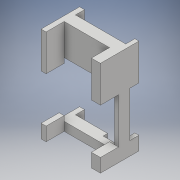
# Autodesk Inventor part: 120mmLaptopStand-Right
Saved by Autodesk Inventor 2017 (Build 210142000, 142)
## iProperties
Created: 2016-09-14
Part Number: 120mmLaptopStand-Right
Material: Generic
Document SubType Name: Modeling
Designer: Schmidty15
Density: 1 g/cm^3
Appearance: Default
Author: Schmidty15
Autodesk Inventor part; units mm, degrees
ref_plane "YZ Plane" through (0, 0, 0) normal (1, 0, 0) x (0, 1, 0)
ref_plane "XZ Plane" through (0, 0, 0) normal (0, 1, 0) x (-1, 0, 0)
ref_plane "XY Plane" through (0, 0, 0) normal (0, 0, 1) x (1, 0, 0)
sketch "Sketch1" plane through (0, 0, 0) normal (0, 1, 0) x (-1, 0, 0)
  point P0 (0, 0)
sketch "Sketch2" plane through (0, 0, 0) normal (0, 1, 0) x (-1, 0, 0)
  line L0 (0, 0) -> (-160, 0)
  line L1 (-160, 0) -> (-160, 210)
  line L2 (-160, 210) -> (0, 210)
  line L3 (0, 210) -> (0, 0)
  dimension "d0" = 160
  dimension "d1" = 210
  constraints: 8 end point, 2 parallel, 1 horizontal, 1 perpendicular
  measures "d0" distance of L1.end L2.end
  measures "d1" distance of L0.end L1.end
extrude "Extrusion1" add sketch "Sketch2" against normal blind 55
sketch "Sketch3" plane through (0, 0, 0) normal (-1, 0, 0) x (0, 0, 1)
  line L0 (0, 0) -> (0, -55) projected
  line L1 (0, 0) -> (9, 0)
  line L2 (9, 0) -> (9, -10)
  line L3 (9, -10) -> (0, -10)
  line L4 (0, -10) -> (0, 0)
  line L5 (0, 0) -> (210, 0) projected
  line L6 (9, -10) -> (131, -10)
  line L7 (131, -10) -> (131, 0)
  line L8 (131, 0) -> (9, 0)
  line L9 (9, 0) -> (9, -10)
  dimension "d4" = 9
  dimension "d5" = 10
  dimension "d6" = 122
  constraints: 16 end point, 4 parallel, 2 horizontal, 2 perpendicular, 1 point on line
  measures "d4" distance of L2.end L3.end
  measures "d5" distance of L1.end L2.end
  measures "d6" distance of L8.end L7.end
extrude "Extrusion2" cut sketch "Sketch3" against normal blind 122 contours L5 L7 L6 L2
sketch "Sketch4" plane through (160, 0, 210) normal (1, 0, 0) x (0, 0, -1)
  line L0 (210, 0) -> (210, -55) projected
  line L1 (210, -55) -> (0, -55)
  line L2 (0, -55) -> (0, 0)
  line L3 (0, 0) -> (210, 0)
  line L4 (210, 0) -> (210, -55)
  constraints: 8 end point, 2 parallel, 1 horizontal, 1 perpendicular
extrude "Extrusion3" cut sketch "Sketch4" against normal blind 29
sketch "Sketch5" plane through (0, -10, 131) normal (0, 1, 0) x (1, 0, 0)
  line L0 (122, 122) -> (122, 0) projected
  line L1 (0, 122) -> (122, 122)
  line L2 (122, 122) -> (122, 0)
  line L3 (122, 0) -> (0, 0)
  line L4 (0, 0) -> (0, 122)
  point P0 (0, 131)
  constraints: 8 end point, 2 parallel, 1 horizontal, 1 perpendicular
extrude "Extrusion4" cut sketch "Sketch5" against normal blind 25
sketch "Sketch6" plane through (0, -35, 131) normal (0, 1, 0) x (1, 0, 0)
  line L0 (0, 122) -> (122, 122) projected
  line L1 (0, 122) -> (11, 122)
  line L2 (11, 122) -> (11, 111)
  line L3 (11, 111) -> (0, 111)
  line L4 (0, 111) -> (0, 122)
  line L5 (122, 122) -> (122, 0) projected
  line L6 (122, 122) -> (111, 122)
  line L7 (111, 122) -> (111, 111)
  line L8 (111, 111) -> (122, 111)
  line L9 (122, 111) -> (122, 122)
  line L10 (11, 111) -> (111, 111)
  line L11 (111, 111) -> (111, 11)
  line L12 (111, 11) -> (11, 11)
  line L13 (11, 11) -> (11, 111)
  point P0 (0, 131)
  dimension "d13" = 11
  dimension "d14" = 11
  dimension "d15" = 11
  dimension "d16" = 11
  dimension "d17" = 100
  constraints: 24 end point, 6 parallel, 3 horizontal, 3 perpendicular, 1 point on line
  measures "d13" distance of L2.end L3.end
  measures "d14" distance of L1.end L2.end
  measures "d15" distance of L8.end L7.end
  measures "d16" distance of L7.end L6.end
  measures "d17" distance of L10.end L11.end
extrude "Extrusion5" cut sketch "Sketch6" against normal blind 20 contours L10 L11 L12 L13
sketch "Sketch7" plane through (0, -35, 131) normal (0, 1, 0) x (1, 0, 0)
  line L0 (11, 11) -> (11, 111) projected
  line L1 (0, 122) -> (122, 122) projected
  line L2 (11, 111) -> (111, 111)
  line L3 (111, 111) -> (111, 122)
  line L4 (111, 122) -> (11, 122)
  line L5 (11, 122) -> (11, 111)
  line L6 (0, 0) -> (0, 122) projected
  line L7 (11, 111) -> (0, 111)
  line L8 (0, 111) -> (0, 11)
  line L9 (0, 11) -> (11, 11)
  line L10 (11, 11) -> (11, 111)
  line L11 (111, 111) -> (111, 11) projected
  line L12 (122, 122) -> (122, 0) projected
  line L13 (111, 111) -> (122, 111)
  line L14 (122, 111) -> (122, 11)
  line L15 (122, 11) -> (111, 11)
  line L16 (111, 11) -> (111, 111)
  line L17 (111, 11) -> (11, 11) projected
  line L18 (11, 11) -> (111, 11)
  line L19 (111, 11) -> (111, 0)
  line L20 (111, 0) -> (11, 0)
  line L21 (11, 0) -> (11, 11)
  point P0 (0, 131)
  dimension "d20" = 100
  dimension "d21" = 100
  dimension "d22" = 100
  dimension "d23" = 11
  constraints: 32 end point, 8 parallel, 4 horizontal, 4 perpendicular, 4 point on line
  measures "d20" distance of L4.end L3.end
  measures "d21" distance of L8.end L7.end
  measures "d22" distance of L19.end L20.end
  measures "d23" distance of L18.end L19.end
extrude "Extrusion6" cut sketch "Sketch7" against normal blind 20 contours L9 L6 L7 L0 | L17 L19 L20 L21 | L5 L1 L3 L2 | L11 L13 L12 L15
sketch "Sketch8" plane through (0, 0, 0) normal (0, 1, 0) x (1, 0, 0)
  line L0 (0, 0) -> (131, 0) projected
  line L1 (0, -9) -> (122, -9) projected
  line L2 (131, 0) -> (111, 0)
  line L3 (111, 0) -> (111, -9)
  line L4 (111, -9) -> (131, -9)
  line L5 (131, -9) -> (131, 0)
  line L6 (111, 0) -> (11, 0)
  line L7 (11, 0) -> (11, -9)
  line L8 (11, -9) -> (111, -9)
  line L9 (111, -9) -> (111, 0)
  line L10 (131, -9) -> (122, -9)
  line L11 (122, -9) -> (122, -119)
  line L12 (122, -119) -> (131, -119)
  line L13 (131, -119) -> (131, -9)
  dimension "d26" = 20
  dimension "d27" = 100
  dimension "d28" = 9
  dimension "d29" = 110
  constraints: 24 end point, 6 parallel, 3 horizontal, 3 perpendicular, 2 point on line
  measures "d26" distance of L4.end L3.end
  measures "d27" distance of L8.end L7.end
  measures "d28" distance of L12.end L11.end
  measures "d29" distance of L11.end L10.end
extrude "Extrusion7" cut sketch "Sketch8" against normal blind 10 contours L0 L3 L1 L7 | L13 L12 L11 L4
sketch "Sketch10" plane through (0, -35, 9) normal (0, 0, 1) x (1, 0, 0)
  line L0 (111, 35) -> (131, 35) projected
  line L1 (131, 35) -> (122, 35)
  line L2 (122, 35) -> (122, 25)
  line L3 (122, 25) -> (131, 25)
  line L4 (131, 25) -> (131, 35)
  point P0 (0, 35)
  constraints: 8 end point, 2 parallel, 1 horizontal, 1 perpendicular
extrude "Extrusion8" add sketch "Sketch10" along normal blind 11
sketch "Sketch11" plane through (122, 0, 131) normal (0, 0, -1) x (-1, 0, 0)
  line L0 (0, 0) -> (122, 0) projected
  line L1 (0, 0) -> (111, 0)
  line L2 (111, 0) -> (111, -10)
  line L3 (111, -10) -> (0, -10)
  line L4 (0, -10) -> (0, 0)
  dimension "d38" = 111
  dimension "d39" = 10
  constraints: 8 end point, 2 parallel, 1 horizontal, 1 perpendicular
  measures "d38" distance of L2.end L3.end
  measures "d39" distance of L1.end L2.end
extrude "Extrusion9" cut sketch "Sketch11" against normal blind 80
sketch "Sketch12" plane through (0, -55, 210) normal (0, 0, 1) x (1, 0, 0)
  line L0 (122, 45) -> (11, 45) projected
  line L1 (11, 45) -> (11, 20)
  line L2 (131, 0) -> (0, 0) projected
  line L3 (11, 20) -> (111, 20)
  line L4 (111, 20) -> (111, 0)
  line L5 (111, 0) -> (11, 0)
  line L6 (11, 0) -> (11, 20)
  point P0 (0, 55)
  dimension "d42" = 25
  dimension "d43" = 100
  constraints: 10 end point, 2 parallel, 1 horizontal, 1 perpendicular, 1 point on line, 1 vertical
  measures "d42" distance of L0.end L1.end
  measures "d43" distance of L4.end L5.end
extrude "Extrusion10" cut sketch "Sketch12" against normal blind 220
sketch "Sketch13" plane through (122, 0, 0) normal (-1, 0, 0) x (0, 0, 1)
  line L0 (0, -55) -> (210, -55) projected
  line L1 (20, -35) -> (120, -35)
  line L2 (120, -35) -> (120, -55)
  line L3 (120, -55) -> (20, -55)
  line L4 (20, -55) -> (20, -35)
  point P0 (0, 0)
  dimension "d46" = 100
  constraints: 8 end point, 2 parallel, 1 horizontal, 1 perpendicular, 1 point on line
  measures "d46" distance of L2.end L3.end
extrude "Extrusion11" cut sketch "Sketch13" against normal blind 9
sketch "Sketch14" plane through (0, -35, 9) normal (0, 0, 1) x (1, 0, 0)
  line L0 (0, 35) -> (11, 35) projected
  line L1 (0, 35) -> (11, 35)
  line L2 (11, 35) -> (11, 0)
  line L3 (11, 0) -> (0, 0)
  line L4 (0, 0) -> (0, 35)
  line L5 (111, 25) -> (11, 25) projected
  line L6 (111, 0) -> (122, 0) projected
  line L7 (11, 25) -> (122, 25)
  line L8 (122, 25) -> (122, 0)
  line L9 (122, 0) -> (11, 0)
  line L10 (11, 0) -> (11, 25)
  line L11 (111, 25) -> (111, 35) projected
  line L12 (111, 35) -> (122, 35)
  line L13 (122, 35) -> (122, 25)
  line L14 (122, 25) -> (111, 25)
  line L15 (111, 25) -> (111, 35)
  constraints: 24 end point, 6 parallel, 3 horizontal, 3 perpendicular
sketch "Sketch15" plane through (0, -35, 20) normal (0, 0, 1) x (1, 0, 0)
  line L0 (11, 0) -> (11, -20) projected
  line L1 (0, -20) -> (11, -20)
  line L2 (11, -20) -> (11, 0)
  line L3 (11, 0) -> (0, 0)
  line L4 (0, 0) -> (0, -20)
  line L5 (131, 0) -> (131, -20) projected
  line L6 (111.5686, -20) -> (131, -20)
  line L7 (131, -20) -> (131, 0)
  line L8 (131, 0) -> (111.5686, 0)
  line L9 (122, 35) -> (122, 25) projected
  line L10 (131, 25) -> (122, 25) projected
  line L11 (122, 35) -> (131, 35)
  line L12 (131, 35) -> (131, 25)
  line L13 (131, 25) -> (122, 25)
  line L14 (122, 25) -> (122, 35)
  line L15 (111, 0) -> (111, -20) projected
  line L16 (111, 0) -> (131, 0)
  line L17 (131, 0) -> (131, -20)
  line L18 (131, -20) -> (111, -20)
  line L19 (111, -20) -> (111, 0)
  point P0 (0, 35)
  constraints: 30 end point, 7 parallel, 4 horizontal, 4 perpendicular, 1 point on line
extrude "Extrusion12" add sketch "Sketch14" along normal blind 10
extrude "Extrusion13" add sketch "Sketch15" along normal blind 10
sketch "Sketch16" plane through (0, -35, 131) normal (0, 0, -1) x (-1, 0, 0)
  line L0 (-11, 35) -> (-11, 25) projected
  line L1 (-11, 0) -> (0, 0) projected
  line L2 (-11, 35) -> (0, 35)
  line L3 (0, 35) -> (0, 0)
  line L4 (0, 0) -> (-11, 0)
  line L5 (-11, 0) -> (-11, 35)
  line L6 (-11, 25) -> (-122, 25) projected
  line L7 (-122, 25) -> (-122, 0) projected
  line L8 (-11, 25) -> (-122, 25)
  line L9 (-122, 25) -> (-122, 0)
  line L10 (-122, 0) -> (-11, 0)
  line L11 (-11, 0) -> (-11, 25)
  constraints: 16 end point, 4 parallel, 2 horizontal, 2 perpendicular
extrude "Extrusion14" cut sketch "Sketch16" against normal blind 10
sketch "Sketch18" plane through (131, -55, 120) normal (0, 0, -1) x (-1, 0, 0)
  line L0 (0, 0) -> (0, 20) projected
  line L1 (9, 20) -> (20, 20) projected
  line L2 (0, 0) -> (20, 0)
  line L3 (20, 0) -> (20, 20)
  line L4 (20, 20) -> (0, 20)
  line L5 (0, 20) -> (0, 0)
  line L6 (120, 20) -> (120, 0) projected
  line L7 (131, 20) -> (131, 0) projected
  line L8 (120, 0) -> (131, 0)
  line L9 (131, 0) -> (131, 20)
  line L10 (131, 20) -> (120, 20)
  line L11 (120, 20) -> (120, 0)
  point P0 (131, 55)
  constraints: 16 end point, 4 parallel, 2 horizontal, 2 perpendicular
extrude "Extrusion15" cut sketch "Sketch18" against normal blind 10
sketch "Sketch19" plane through (131, 0, 119) normal (0, 0, -1) x (-1, 0, 0)
  line L0 (0, -10) -> (9, -10) projected
  line L1 (9, -10) -> (0, -10)
  line L2 (0, -10) -> (0, 0)
  line L3 (0, 0) -> (9, 0)
  line L4 (9, 0) -> (9, -10)
  point P0 (131, 0)
  constraints: 8 end point, 2 parallel, 1 horizontal, 1 perpendicular
extrude "Extrusion16" cut sketch "Sketch19" against normal blind 11
sketch "Sketch20" plane through (0, -35, 19) normal (0, 0, 1) x (1, 0, 0)
  line L0 (11, 25) -> (111, 25) projected
  line L1 (111, 25) -> (92, 25)
  line L2 (92, 25) -> (92, 15)
  line L3 (92, 15) -> (111, 15)
  line L4 (111, 15) -> (111, 25)
  point P0 (0, 35)
  dimension "d59" = 19
  dimension "d60" = 10
  constraints: 8 end point, 2 parallel, 1 horizontal, 1 perpendicular
  measures "d59" distance of L3.end L2.end
  measures "d60" distance of L2.end L1.end
extrude "Extrusion17" cut sketch "Sketch20" against normal blind 19
sketch "Sketch21" plane through (92, -20, 19) normal (1, 0, 0) x (0, 0, -1)
  line L0 (0, 0) -> (0, 10) projected
  line L1 (19, 10) -> (19, 0) projected
  line L2 (0, 0) -> (19, 0)
  line L3 (19, 0) -> (19, 10)
  line L4 (19, 10) -> (0, 10)
  line L5 (0, 10) -> (0, 0)
  point P0 (19, 20)
  constraints: 8 end point, 2 parallel, 1 horizontal, 1 perpendicular
extrude "Extrusion18" cut sketch "Sketch21" against normal blind 10
sketch "Sketch22" plane through (0, -55, 0) normal (0, -1, 0) x (1, 0, 0)
  line L0 (11, 210) -> (0, 210) projected
  line L1 (11, 141) -> (11, 130) projected
  line L2 (0, 210) -> (11, 210)
  line L3 (11, 210) -> (11, 130)
  line L4 (11, 130) -> (0, 130)
  line L5 (0, 130) -> (0, 210)
  line L6 (11, 210) -> (111, 210) projected
  line L7 (131, 130) -> (131, 210) projected
  line L8 (111, 210) -> (131, 210)
  line L9 (131, 210) -> (131, 130)
  line L10 (131, 130) -> (111, 130)
  line L11 (111, 130) -> (111, 210)
  line L12 (0, 30) -> (0, 19) projected
  line L13 (11, 19) -> (11, 0) projected
  line L14 (0, 30) -> (11, 30)
  line L15 (11, 30) -> (11, 0)
  line L16 (11, 0) -> (0, 0)
  line L17 (0, 0) -> (0, 30)
  line L18 (131, 30) -> (131, 0) projected
  line L19 (111, 30) -> (131, 30)
  line L20 (131, 30) -> (131, 0)
  line L21 (131, 0) -> (111, 0)
  line L22 (111, 0) -> (111, 30)
  constraints: 32 end point, 8 parallel, 4 horizontal, 4 perpendicular
extrude "Extrusion19" add sketch "Sketch22" along normal blind 20
sketch "Sketch23" plane through (0, 0, 0) normal (0, 1, 0) x (1, 0, 0)
  line L0 (0, 0) -> (11, 0) projected
  line L1 (11, -19) -> (11, 0) projected
  line L2 (0, 0) -> (11, 0)
  line L3 (11, 0) -> (11, -19)
  line L4 (11, -19) -> (0, -19)
  line L5 (0, -19) -> (0, 0)
  line L6 (111, 0) -> (111, -19) projected
  line L7 (122, -19) -> (122, -30) projected
  line L8 (111, 0) -> (122, 0)
  line L9 (122, 0) -> (122, -19)
  line L10 (122, -19) -> (111, -19)
  line L11 (111, -19) -> (111, 0)
  line L12 (131, -30) -> (131, 0) projected
  line L13 (122, -30) -> (131, -30)
  line L14 (131, -30) -> (131, 0)
  line L15 (131, 0) -> (122, 0)
  line L16 (122, 0) -> (122, -30)
  line L17 (122, -130) -> (122, -210) projected
  line L18 (131, -210) -> (131, -130) projected
  line L19 (122, -130) -> (131, -130)
  line L20 (131, -130) -> (131, -210)
  line L21 (131, -210) -> (122, -210)
  line L22 (122, -210) -> (122, -130)
  line L23 (11, -210) -> (11, -141) projected
  line L24 (0, -141) -> (11, -141)
  line L25 (11, -141) -> (11, -210)
  line L26 (11, -210) -> (0, -210)
  line L27 (0, -210) -> (0, -141)
  constraints: 40 end point, 10 parallel, 5 horizontal, 5 perpendicular
extrude "Extrusion20" add sketch "Sketch23" along normal blind 10
body "Solid1"
